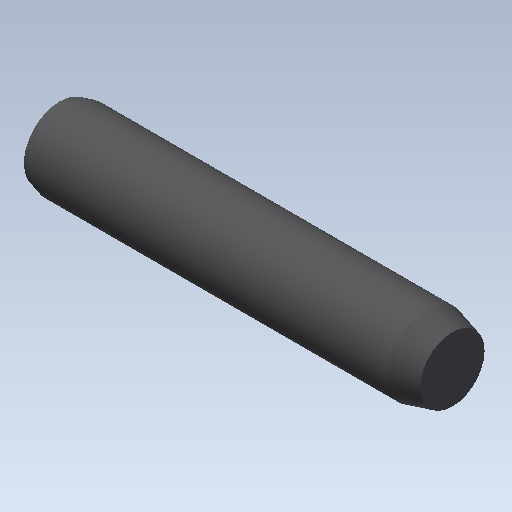
# Autodesk Inventor part: MSVC3-15
Saved by Autodesk Inventor 2020 (Build 240168000, 168)
## iProperties
Created: 2016-12-07
Part Number: MSVC3-15
Catalog Web Link: www.cadenas.de
Description: MSV, MSVC-Dowel Pins - High Precision
Vendor: MISUMI
Document SubType Name: Modeling
Designer: psAdmin
Manufacturer: MISUMI
Mass: 0.104535 g
Surface Area: 1.51412 cm^2
Volume: 0.104535 cm^3
Density: 1 g/cm^3
Material: Generic
Appearance: PSOLRGB-175-175-175
Category: PARTsolutions
Company: MISUMI
PSOL_IDENT_0: {$CADENAS_DATA\23d-libs\misumi\metric\28_keys_magnets\msv.prj},155 {VTYP=3D},{NB=MSVC3-15},{LINA=MSV
PSOL_IDENT_1: C3-15},{NN=MSV, MSVC},{DATE=17.06.2016 05:51:05},{GEOMDATE=31.01.2012},{VERSION=},{LINEID=20},{LINES
PSOL_IDENT_2: UBID=-1},{WBVAR=D,L}  {NB=MSVC3-15},{LINA=MSVC3-15},{KT=DUMMY},{PN=MSVC3-15},{TYPE=MSVC},{MAT=440C S
PSOL_IDENT_3: tainless Steel},{HARD=58HRC~},{D=3.0},{DALG=[1,1.5,2,3,4,5,6,8,10]},{L=15},{LALG=[6,8,10,15,20,25,30
PSOL_IDENT_4: ]},{LL1=1.0},{LL2=0.5}
NN: MSV, MSVC
NT: Dowel Pins - High Precision
NB: MSVC3-15
NBSYN: $PN.
LINA: MSVC3-15
PN: MSVC3-15
MAT: 440C Stainless Steel
HARD: 58HRC~
D: 3.0
L: 15
LL1: 1.0
LL2: 0.5
SUPPLIER: MISUMI
ARTICLENO: MSVC3-15
BOMINFO: MSVC3-15
CREATOR: CADENAS GmbH
Title: MSVC3-15
Author: Cadenas PARTsolutions
Comments: Dowel Pins - High Precision
Autodesk Inventor part; units mm, degrees
ref_plane "YZ Plane" through (0, 0, 0) normal (1, 0, 0) x (0, 1, 0)
ref_plane "XZ Plane" through (0, 0, 0) normal (0, 1, 0) x (-1, 0, 0)
ref_plane "XY Plane" through (0, 0, 0) normal (0, 0, 1) x (1, 0, 0)
sketch "Sketch_1" plane through (0, 0, 0) normal (0, 0, 1) x (1, 0, 0)
  line L0 (7.5, 0) -> (-7.5, 0)
  line L1 (-7.5, 0) -> (-7.5, 1.366)
  line L2 (-7.5, 1.366) -> (-7, 1.5)
  line L3 (-7, 1.5) -> (6.5, 1.5)
  line L4 (6.5, 1.5) -> (7.5, 1.2321)
  line L5 (7.5, 1.2321) -> (7.5, 0)
  line L6 (7.5, 0) -> (-7.5, 0)
  constraints: 14 end point
revolve "Revolution1" add sketch "Sketch_1" angle 360 about axis through (7.5, 0, 0) along (1, 0, 0)
body "Solid1"
